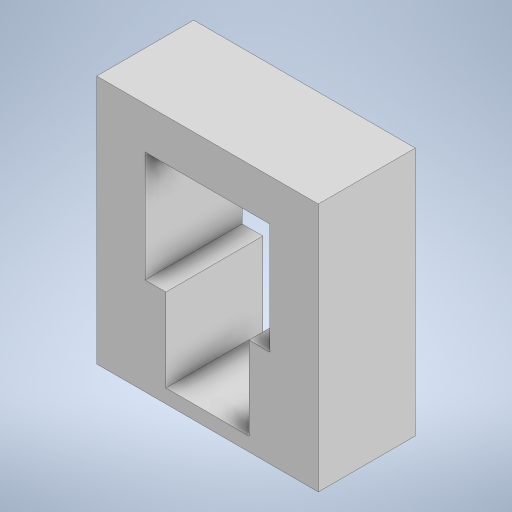
# Autodesk Inventor part: BT002_Matrize
Saved by Autodesk Inventor 2023 (Build 270158000, 158)
## iProperties
Created: 2022-04-24
Part Number: BT002_Matrize
Material: Generic
Document SubType Name: Modeling
Designer: Altar
Density: 1 g/cm^3
Appearance: Default
Author: Altar
Autodesk Inventor part; units mm, degrees
ref_plane "YZ Plane" through (0, 0, 0) normal (1, 0, 0) x (0, 1, 0)
ref_plane "XZ Plane" through (0, 0, 0) normal (0, 1, 0) x (-1, 0, 0)
ref_plane "XY Plane" through (0, 0, 0) normal (0, 0, 1) x (1, 0, 0)
sketch "Sketch1" plane through (0, 0, 0) normal (0, 0, 1) x (1, 0, 0)
  line L0 (-11.5482, -7.036) -> (-11.5482, 82.964)
  line L1 (-11.5482, 82.964) -> (68.4518, 82.964)
  line L2 (68.4518, 82.964) -> (68.4518, -7.036)
  line L3 (68.4518, -7.036) -> (-11.5482, -7.036)
  line L4 (5.9518, 27.964) -> (5.9518, 67.964)
  line L5 (5.9518, 67.964) -> (50.9518, 67.964)
  line L6 (50.9518, 67.964) -> (50.9518, 27.964)
  line L7 (50.9518, 27.964) -> (43.4518, 27.964)
  line L8 (43.4518, 27.964) -> (43.4518, -2.036)
  line L9 (43.4518, -2.036) -> (13.4518, -2.036)
  line L10 (13.4518, -2.036) -> (13.4518, 27.964)
  line L11 (13.4518, 27.964) -> (5.9518, 27.964)
  point P0 (0, 0)
  dimension "d0" = 90
  dimension "d1" = 80
  dimension "d2" = 90
  dimension "d3" = 45
  dimension "d4" = 40
  dimension "d5" = 7.5
  dimension "d6" = 30
  dimension "d7" = 17.5
  dimension "d8" = 15
  dimension "d9" = 30
  constraints: 24 end point, 9 perpendicular, 2 vertical, 1 point on line
  measures "d0" distance of L0.start L0.end
  measures "d1" distance of L0.end L1.end
  measures "d2" distance of L1.end L2.end
  measures "d3" distance of L4.end L5.end
  measures "d4" distance of L5.end L6.end
  measures "d5" distance of L6.end L7.end
  measures "d6" distance of L8.end L9.end
  measures "d7" distance between parallel lines of L0 L4
  measures "d8" distance between parallel lines of L1 L5
  measures "d9" distance of L7.end L8.end
extrude "Extrusion1" add sketch "Sketch1" against normal blind 35
body "Solid1"
